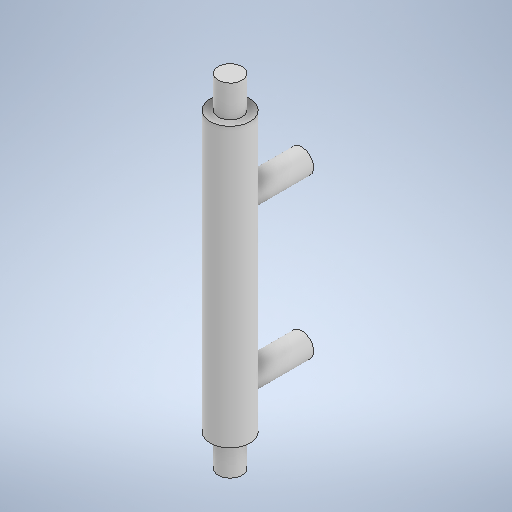
# Autodesk Inventor part: verbindung2
Saved by Autodesk Inventor 2025.1 (Build 291241000, 241)
## iProperties
Created: 2024-08-07
Part Number: verbindung2
Material: Generisch
Document SubType Name: Modeling
Designer: ffogue
Density: 1 g/cm^3
Appearance: Vorgabe
Author: ffogue
Autodesk Inventor part; units mm, degrees
ref_plane "YZ Plane" through (0, 0, 0) normal (1, 0, 0) x (0, 1, 0)
ref_plane "XY Plane" through (0, 0, 0) normal (0, 0, 1) x (1, 0, 0)
sketch "Sketch1" plane through (0, 0, 0) normal (0, 0, 1) x (1, 0, 0)
  circle A0 centre (0, 0) radius 5
  dimension "d0" = 10
  constraints: 1 centre point, 1 coincident
  measures "d0" diameter of A0
extrude "Extrusion1" add sketch "Sketch1" along normal blind 70
sketch "Sketch2" plane through (0, 0, 70) normal (0, 0, 1) x (1, 0, 0)
  circle A0 centre (0, 0) radius 3
  dimension "d3" = 6
  constraints: 1 centre point, 1 coincident
  measures "d3" diameter of A0
extrude "Extrusion2" add sketch "Sketch2" along normal blind 8
sketch "Sketch3" plane through (0, 0, 0) normal (0, 0, -1) x (-1, 0, 0)
  circle A0 centre (0, 0) radius 3 projected
  circle A1 centre (0, 0) radius 3
  dimension "d6" = 6
  constraints: 1 centre point, 1 coincident
  measures "d6" diameter of A1
extrude "Extrusion3" add sketch "Sketch3" along normal blind 8
ref_plane "Work Plane1" through (0, 18, 0) normal (0, 1, 0) x (-1, 0, 0)
sketch "Sketch4" plane through (0, 18, 0) normal (0, 1, 0) x (-1, 0, 0)
  circle A0 centre (0, 10) radius 3
  circle A1 centre (0, 50) radius 3
  line L0 (5, 0) -> (5, 70) projected
  line L1 (5, 35) -> (17.3974, 35) construction
  point P0 (0, 0)
  dimension "d10" = 6
  dimension "d11" = 6
  dimension "d12" = 40
  dimension "d13" = 10
  constraints: 2 centre point, 2 end point, 2 vertical alignment, 1 horizontal, 1 midpoint
  measures "d10" diameter of A0
  measures "d11" diameter of A1
  measures "d12" distance of A1.centre A0.centre
  measures "d13" distance of point (0, 0) A0.centre
extrude "Extrusion4" add sketch "Sketch4" against normal up to surface
body "Solid1"
